Autodesk Fusion 360 part; units mm, degrees
(part 2 of 2)
  constraint tangent L242 A245
  constraint tangent L236 A246
  constraint tangent L247 A246
  constraint tangent L236 A247
  constraint tangent L248 A247
  constraint tangent L235 A248
  constraint tangent L247 A248
  constraint tangent L234 A249
  constraint tangent L242 A249
  constraint tangent L237 A250
  constraint tangent L248 A250
  constraint tangent L237 A251
  constraint tangent L249 A251
  constraint tangent L238 A252
  constraint tangent L249 A252
  constraint tangent L228 A253
  constraint tangent L243 A253
  constraint tangent L229 A254
  constraint tangent L244 A254
  constraint tangent L230 A255
  constraint tangent L241 A255
  constraint tangent L230 A256
  constraint tangent L245 A256
  constraint tangent L231 A257
  constraint tangent L246 A257
  constraint coincident L215 L107.start
  constraint coincident L216 L106.start
  constraint perpendicular L216 L250
  constraint perpendicular L233 L251
  constraint collinear L252 L253
  constraint collinear L254 L255
  constraint tangent L250 A258
  constraint tangent L253 A258
  constraint tangent L250 A259
  constraint tangent L254 A259
  constraint tangent L251 A260
  constraint tangent L252 A260
  constraint tangent L251 A261
  constraint tangent L255 A261
  constraint concentric A111 A262
  constraint concentric A112 A263
  constraint tangent L109 A264
  constraint tangent L109 A265
  constraint tangent A266 L256
  constraint tangent L108 A267
  constraint tangent L256 A267
  constraint tangent L108 A268
  measures "d1" diameter of A0
  measures "d2" diameter of A1
  measures "d3" diameter of A2
  measures "d4" diameter of A3
  measures "d5" diameter of A4
  measures "d9" diameter of A111
  measures "d12" diameter of A112
  measures "d305" diameter of A262
  measures "d306" diameter of A263
extrude "Extrude1" add sketch "mriya-bumper-sla" along normal blind 10.5 contours L106 L107 L215 A223 L216 L232 L233 A239 | L106 L107 L206 A214 L207 A215 L208 A216 L209 A217 L210 A218 L211 A219 L212 A220 L213 A221 L214 A222 L215 L216 A224 L217 A225 L218 A226 L219 A227 L220 A228 L221 A229 L222 A230 L223 A231 L224 A232 L225 A233 L226 A234 L227 A235 L228 L229 L230 L231 L232 L233 L234 L235 L236 L237 L238 L239 L240 L241 L242 L243 L244 L245 L246 L247 L248 L249 A236 A237 A238 A240 A241 A242 A243 A244 A245 A246 A247 A248 A249 A250 A251 A252 A253 A254 A255 A256 A257 makes body 1
extrude "Extrude2" add sketch "mriya-bumper-sla" along normal blind 17 contours L106 L107 L215 A223 L216 L232 L233 A239 bodies 1
extrude "Extrude3" add sketch "mriya-bumper-sla" along normal blind 2 from surface at 1.7 contours L108 L109 L206 A214 L207 A215 L208 A216 L209 A217 L210 A218 L211 A219 L212 A220 L213 A221 L214 A222 L215 L216 A224 L217 A225 L218 A226 L219 A227 L220 A228 L221 A229 L222 A230 L223 A231 L224 A232 L225 A233 L226 A234 L227 A235 A264 A265 A266 L256 A267 A268 | L109 L216 A264 A265 | L108 L215 A223 L216 A266 L256 A267 A268 | A114 | A115 | A116 | A117 | A262 | A263 bodies 1
extrude "Extrude6" add sketch "mriya-bumper-sla" along normal blind 1 from surface at 14.3 contours L108 L215 A223 L216 A266 L256 A267 A268 bodies 1
extrude "Extrude14" add sketch "mriya-bumper-sla" along normal blind 1 from surface at 7.7 contours L109 L216 A264 A265 bodies 1
chamfer "Chamfer5" distance 0.599 angle 45 4 edges at (-14.85, 78.0932, 14.3) (-7.4686, 77.6246, 14.3) (-7, 58.2443, 14.3) (-7, 9.5932, 7.7) on bodies 1
sketch "power-switch" plane through (-4.5, 0, 0) normal (1, 0, 0) x (0, 1, 0)
  line L0 (1.9932, 0) -> (76.4932, 0)
  line L1 (76.4932, 0) -> (76.4932, 17)
  line L2 (76.4932, 17) -> (19.2932, 17)
  line L3 (19.2932, 17) -> (19.2932, 10.5)
  line L4 (19.2932, 10.5) -> (1.9932, 10.5)
  line L5 (1.9932, 10.5) -> (1.9932, 0)
  line L6 (36.0432, 5.45) -> (25.7432, 5.45)
  line L7 (25.7432, 5.45) -> (25.7432, 8.25)
  line L8 (25.7432, 8.25) -> (36.0432, 8.25)
  line L9 (36.0432, 8.25) -> (36.0432, 5.45)
  line L10 (37.3932, 3.1) -> (24.3932, 3.1)
  line L11 (23.3932, 4.1) -> (23.3932, 9.6)
  line L12 (24.3932, 10.6) -> (37.3932, 10.6)
  line L13 (38.3932, 9.6) -> (38.3932, 4.1)
  arc A0 (24.3932, 10.6) -> (23.3932, 9.6) centre (24.3932, 9.6) ccw
  arc A1 (38.3932, 9.6) -> (37.3932, 10.6) centre (37.3932, 9.6) ccw
  arc A2 (37.3932, 3.1) -> (38.3932, 4.1) centre (37.3932, 4.1) ccw
  arc A3 (23.3932, 4.1) -> (24.3932, 3.1) centre (24.3932, 4.1) ccw
  line L14 (19.2932, 10.5) -> (1.8932, 10.5)
  line L15 (1.8932, 10.5) -> (1.8932, 0)
  line L16 (1.8932, 0) -> (76.5932, 0)
  line L17 (76.5932, 0) -> (76.5932, 17)
  line L18 (76.5932, 17) -> (19.2932, 17)
  line L19 (19.2932, 17) -> (19.2932, 10.5)
  constraint perpendicular L6 L7
  constraint tangent L11 A0
  constraint tangent L12 A0
  constraint tangent L12 A1
  constraint tangent L13 A1
  constraint tangent L10 A2
  constraint tangent L13 A2
  constraint tangent L10 A3
  constraint tangent L11 A3
  constraint vertical L7
  constraint perpendicular L7 L8
  constraint vertical L9
extrude "Extrude8" cut sketch "power-switch" against normal blind 2.5 contours L6 L7 L8 L9 bodies 1
extrude "Extrude9" cut sketch "power-switch" against normal blind 1 contours L10 L11 L12 L13 A0 A1 A2 A3 bodies 1
fillet "Fillet23" radius 0.1 8 edges at (-4.5, 23.3932, 6.85) (-4.5, 23.6861, 10.3071) (-4.5, 30.8932, 10.6) (-4.5, 38.1003, 10.3071) (-4.5, 38.3932, 6.85) (-4.5, 38.1003, 3.3929) (-4.5, 30.8932, 3.1) (-4.5, 23.6861, 3.3929) on bodies 1
fillet "Fillet24" radius 1 8 edges at (-5.5, 30.8932, 3.1) (-5.5, 23.6861, 3.3929) (-5.5, 23.3932, 6.85) (-5.5, 23.6861, 10.3071) (-5.5, 30.8932, 10.6) (-5.5, 38.1003, 10.3071) (-5.5, 38.3932, 6.85) (-5.5, 38.1003, 3.3929) on bodies 1
chamfer "Chamfer4" distance 0.5 angle 45 4 edges at (-7, 30.8932, 5.45) (-7, 36.0432, 6.85) (-7, 30.8932, 8.25) (-7, 25.7432, 6.85) on bodies 1
sketch "usb-c" plane through (0, 80.5932, 0) normal (0, 1, 0) x (-1, 0, 0)
  line L0 (8.5, 0) -> (41.1088, 0)
  line L1 (41.1088, 0) -> (41.1088, 10.5)
  line L2 (41.1088, 10.5) -> (25.8, 10.5)
  line L3 (25.8, 10.5) -> (25.8, 17)
  line L4 (25.8, 17) -> (8.5, 17)
  line L5 (8.5, 17) -> (8.5, 0)
  line L6 (10.1002, 11.2) -> (10.1002, 10)
  arc A0 (21.0002, 11.05) -> (19.7002, 12.35) centre (19.7002, 11.05) ccw
  arc A1 (11.8003, 10.15) -> (13.1003, 8.85) centre (13.1002, 10.15) ccw
  line L7 (22.7003, 11.2) -> (22.7003, 10)
  line L8 (13.1002, 12.35) -> (19.7002, 12.35)
  line L9 (11.8003, 10.15) -> (11.8003, 11.05)
  arc A2 (10.1002, 10) -> (13.1002, 7) centre (13.1002, 10) ccw
  line L10 (13.1002, 14.2) -> (19.7003, 14.2)
  arc A3 (13.1002, 14.2) -> (10.1002, 11.2) centre (13.1002, 11.2) ccw
  line L11 (19.7003, 7) -> (13.1002, 7)
  arc A4 (19.7003, 7) -> (22.7003, 10) centre (19.7003, 10) ccw
  arc A5 (22.7002, 11.2) -> (19.7003, 14.2) centre (19.7003, 11.2) ccw
  arc A6 (13.1002, 12.35) -> (11.8003, 11.05) centre (13.1002, 11.05) ccw
  line L12 (19.7002, 8.85) -> (13.1002, 8.85)
  line L13 (21.0002, 11.05) -> (21.0002, 10.15)
  arc A7 (19.7002, 8.85) -> (21.0002, 10.15) centre (19.7003, 10.15) ccw
  constraint horizontal L11
  constraint tangent L9 A6
  constraint tangent L8 A6
  constraint tangent A1 L12
  constraint tangent A1 L9
  constraint tangent A0 L8
  constraint tangent A0 L13
  constraint tangent L13 A7
  constraint tangent L12 A7
  constraint parallel L7 L9
  constraint tangent L10 A5
  constraint tangent L7 A5
  constraint tangent L7 A4
  constraint tangent L11 A4
  constraint tangent L6 A3
  constraint tangent L10 A3
  constraint tangent A2 L11
  constraint tangent L6 A2
extrude "Extrude10" cut sketch "usb-c" against normal blind 2.5 contours A0 A1 L8 L9 A6 L12 L13 A7 bodies 1
extrude "Extrude11" cut sketch "usb-c" against normal blind 1.2 contours L6 L7 A2 L10 A3 L11 A4 A5 bodies 1
fillet "Fillet16" radius 1 8 edges at (-10.9789, 79.3932, 13.3213) (-16.4003, 79.3932, 14.2) (-21.8216, 79.3932, 13.3213) (-22.7003, 79.3932, 10.6) (-21.8216, 79.3932, 7.8787) (-16.4003, 79.3932, 7) (-10.9789, 79.3932, 7.8787) (-10.1003, 79.3932, 10.6) on bodies 1
fillet "Fillet20" radius 0.1 8 edges at (-10.1003, 80.5932, 10.6) (-10.9789, 80.5932, 13.3213) (-16.4003, 80.5932, 14.2) (-21.8216, 80.5932, 13.3213) (-22.7003, 80.5932, 10.6) (-21.8216, 80.5932, 7.8787) (-16.4003, 80.5932, 7) (-10.9789, 80.5932, 7.8787) on bodies 1
fillet "Fillet30" radius 0.5 4 edges at (-5.75, 19.2932, 10.5) (-5.75, 19.2932, 17) (-25.8, 79.3432, 10.5) (-25.8, 79.3432, 17) on bodies 1
fillet "Fillet27" radius 1.2 90 edges at (-4.5, 47.9432, 17) (-5.6716, 79.4216, 17) (-17.15, 80.5932, 17) (-33.4544, 80.5932, 10.5) (-41.4915, 80.6693, 10.5) (-42.3069, 81.3771, 10.5) (-43.9334, 82.6268, 10.5) (-51.5908, 82.8932, 10.5) (-58.2915, 82.9693, 10.5) (-60.2069, 84.7771, 10.5) (-62.9334, 87.1268, 10.5) (-73.4, 87.3932, 10.5) (-83.8666, 87.1268, 10.5) (-86.0931, 85.2771, 10.5) (-87.5085, 83.9693, 10.5) (-94.7092, 83.8932, 10.5) (-102.8666, 83.6268, 10.5) (-107.2698, 79.6003, 10.5) (-111.0243, 76.0074, 10.5) (-116.0627, 75.8932, 10.5) (-121.8666, 75.6268, 10.5) (-123.4931, 74.3771, 10.5) (-124.3085, 73.6693, 10.5) (-131.4456, 73.5932, 10.5) (-141.0284, 72.4216, 10.5) (-142.2, 42.8932, 10.5) (-141.0284, 13.3648, 10.5) (-120.4435, 12.1932, 10.5) (-100.9649, 12.5357, 10.5) (-96.4569, 16.5593, 10.5) (-92.76, 20.041, 10.5) (-84.5813, 20.1932, 10.5) (-75.6559, 19.7842, 10.5) (-70.5608, 11.5973, 10.5) (-65.0991, 3.0385, 10.5) (-55.8871, 2.4932, 10.5) (-48.3085, 2.4171, 10.5) (-47.4931, 1.7093, 10.5) (-45.8666, 0.4596, 10.5) (-37.1092, 0.1932, 10.5) (-29.3085, 0.1171, 10.5) (-28.4931, -0.5907, 10.5) (-26.8666, -1.8404, 10.5) (-17.0136, -2.1068, 10.5) (-5.6716, -0.9352, 10.5) (-4.5, 10.5932, 10.5) (-24.8044, 80.5932, 0) (-41.4915, 80.6693, 0) (-42.3069, 81.3771, 0) (-43.9334, 82.6268, 0) (-51.5908, 82.8932, 0) (-58.2915, 82.9693, 0) (-60.2069, 84.7771, 0) (-62.9334, 87.1268, 0) (-73.4, 87.3932, 0) (-83.8666, 87.1268, 0) (-86.0931, 85.2771, 0) (-87.5085, 83.9693, 0) (-94.7092, 83.8932, 0) (-102.8666, 83.6268, 0) (-107.2698, 79.6003, 0) (-111.0243, 76.0074, 0) (-116.0627, 75.8932, 0) (-121.8666, 75.6268, 0) (-123.4931, 74.3771, 0) (-124.3085, 73.6693, 0) (-131.4456, 73.5932, 0) (-141.0284, 72.4216, 0) (-142.2, 42.8932, 0) (-141.0284, 13.3648, 0) (-120.4435, 12.1932, 0) (-100.9649, 12.5357, 0) (-96.4569, 16.5593, 0) (-92.76, 20.041, 0) (-84.5813, 20.1932, 0) (-75.6559, 19.7842, 0) (-70.5608, 11.5973, 0) (-65.0991, 3.0385, 0) (-55.8871, 2.4932, 0) (-48.3085, 2.4171, 0) (-47.4931, 1.7093, 0) (-45.8666, 0.4596, 0) (-37.1092, 0.1932, 0) (-29.3085, 0.1171, 0) (-28.4931, -0.5907, 0) (-26.8666, -1.8404, 0) (-17.0136, -2.1068, 0) (-5.6716, -0.9352, 0) (-4.5, 39.2432, 0) (-5.6716, 79.4216, 0) on bodies 1
extrude "Extrude12" cut sketch "mriya-bumper-sla" along normal blind 1 from surface at 1.7 contours A262 | A263 bodies 1
mirror "Mirror1" about plane through (0, 0, 0) normal (1, 0, 0) of bodies 1 makes body 2
named bodies: "Left", "Right"
